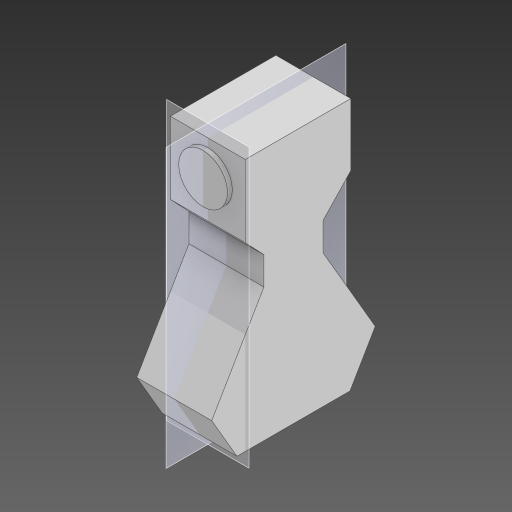
# Autodesk Inventor part: BaseBoundingBox
Saved by Autodesk Inventor 2023 (Build 270158000, 158)
## iProperties
Created: 2023-03-25
Part Number: BaseBoundingBox
Material: Generic
Document SubType Name: Modeling
Designer: Val
Density: 1 g/cm^3
Appearance: Default
Author: Val
Autodesk Inventor part; units mm, degrees
ref_plane "XZ Plane" through (0, 0, 0) normal (0, 1, 0) x (-1, 0, 0)
sketch "Sketch1" plane through (0, 0, 0) normal (1, 0, 0) x (0, 1, 0)
  line L0 (-16, 3.08) -> (16, 3.08)
  line L1 (16, 3.08) -> (16, 0)
  line L2 (16, 0) -> (-16, 0)
  line L3 (-16, 0) -> (-16, 3.08)
  line L4 (-20.328, 3.08) -> (15.75, 3.08) construction
  line L5 (16, 0) -> (-16, 0) construction
  line L6 (-16, 0) -> (-25.6061, 0)
  line L7 (-25.6061, 0) -> (-38.4616, -12.16)
  line L8 (-38.4616, -12.16) -> (-56.7976, -12.16)
  line L9 (-56.7976, -12.16) -> (-115.4254, 21.9603)
  line L10 (-115.4254, 21.9603) -> (-143.8011, 5.4461)
  line L11 (-143.8011, 5.4461) -> (-143.8011, -68.4461)
  line L12 (-143.8011, -68.4461) -> (-115.4254, -84.9603)
  line L13 (-115.4254, -84.9603) -> (-56.7976, -50.84)
  line L14 (-56.7976, -50.84) -> (-38.4616, -50.84)
  line L15 (-38.4616, -50.84) -> (-19.263, -69)
  line L16 (-19.263, -69) -> (21.5, -69)
  line L17 (21.5, -69) -> (21.5, 0)
  line L18 (21.5, 0) -> (16, 0)
  line L19 (-19.5, -69) -> (19.5, -69) construction
  line L20 (-36.9927, -10.7705) -> (-23.8189, 1.6905) construction
  line L21 (-23.8189, -64.6905) -> (-36.9927, -52.2295) construction
  line L22 (-56.7976, -12.16) -> (-40.4836, -12.16) construction
  line L23 (-40.4836, -50.84) -> (-56.7976, -50.84) construction
  line L24 (-133.6344, 11.4742) -> (-125.5921, 15.9321) construction
  line L25 (-125.5921, -78.9321) -> (-133.6344, -74.4742) construction
  point P0 (0, 0)
  point P1 (0, 0)
  point P2 (21.5, -10)
  point P3 (-129.6132, 13.7032)
  point P4 (-129.6132, -76.7032)
  point P5 (16, 0)
  point P6 (16, 0)
  constraints: 34 end point, 7 parallel, 6 collinear, 5 midpoint, 4 perpendicular, 3 point on line, 2 horizontal, 1 coincident, 1 other
extrude "Extrusion3" add sketch "Sketch1" along normal mid plane 49 contours L2 L18 L17 L16 L15 L14 L13 L12 L11 L10 L9 L8 L7 L6
sketch "Sketch3" plane through (-24.5, -25.6061, 0) normal (0, 0, 1) x (1, 0, 0)
  circle A0 centre (24.5, 25.6061) radius 16 projected
extrude "Extrusion4" add sketch "Sketch3" along normal up to surface (3.08 mm away)
body "Solid2"
